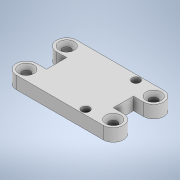
# Autodesk Inventor part: Крепление мотора
Saved by Autodesk Inventor 2020 (Build 240168000, 168)
## iProperties
Created: 2021-05-23
Part Number: Крепление мотора
Material: Типовые
Document SubType Name: Modeling
Designer: Антон
Density: 1 g/cm^3
Appearance: По умолчанию
Author: Антон
Autodesk Inventor part; units mm, degrees
ref_plane "YZ Plane" through (0, 0, 0) normal (1, 0, 0) x (0, 1, 0)
ref_plane "XZ Plane" through (0, 0, 0) normal (0, 1, 0) x (-1, 0, 0)
ref_plane "XY Plane" through (0, 0, 0) normal (0, 0, 1) x (1, 0, 0)
sketch "Эскиз1" plane through (0, 0, 0) normal (0, 1, 0) x (-1, 0, 0)
  line L0 (0, 0) -> (26.5, 0)
  line L1 (26.5, 0) -> (26.5, -24)
  line L2 (26.5, -24) -> (0, -24)
  line L3 (0, -24) -> (0, 0)
  dimension "d0" = 26.5
  dimension "d1" = 24
  constraints: 8 end point, 2 parallel, 1 horizontal, 1 perpendicular
  measures "d0" distance of L1.end L2.end
  measures "d1" distance of L0.end L1.end
extrude "Выдавливание1" add sketch "Эскиз1" along normal blind 5
sketch "Эскиз2" plane through (0, 5, 0) normal (0, 1, 0) x (1, 0, 0)
  line L0 (0, 0) -> (0, 24) projected
  line L1 (0, 12) -> (-5, 12)
  line L2 (-5, 12) -> (-5, 2)
  line L3 (-5, 12) -> (-5, 22)
  dimension "d4" = 5
  dimension "d5" = 10
  constraints: 6 end point, 2 vertical, 1 collinear, 1 midpoint, 1 perpendicular
  measures "d4" distance of L1.start L1.end
  measures "d5" distance of L1.end L2.end
hole "Отверстие1" at (-5, 5, -2) at (-5, 5, -22) direction (0, -1, 0) diameter 3.2 end through all
sketch "Эскиз3" plane through (0, 0, 0) normal (0, -1, 0) x (1, 0, 0)
  line L0 (-26.5, 0) -> (0, 0) projected
  line L1 (0, 0) -> (8, 0)
  line L2 (8, 0) -> (8, -8)
  line L3 (8, -8) -> (0, -8)
  line L4 (0, -8) -> (0, 0)
  dimension "d13" = 8
  dimension "d14" = 8
  constraints: 8 end point, 2 parallel, 1 horizontal, 1 perpendicular
  measures "d13" distance of L2.end L3.end
  measures "d14" distance of L1.end L2.end
extrude "Выдавливание2" add sketch "Эскиз3" against normal blind 5
sketch "Эскиз4" plane through (0, 5, 0) normal (0, 1, 0) x (1, 0, 0)
  line L0 (8, 8) -> (0, 8) projected
  line L1 (4, 8) -> (4, 0)
  point P0 (0, 0)
  point P1 (4, 4)
  constraints: 2 end point, 2 midpoint, 1 vertical
hole "Отверстие2" at (4, 5, -4) direction (0, -1, 0) diameter 3.2 end through all countersink diameter 6 countersink angle 90
fillet "Сопряжение1" radius 4 2 edges at (8, 2.5, 0) (8, 2.5, -8)
ref_plane "РабПлоскость1" through (-26.5, 0, -12) normal (0, 0, 1) x (1, 0, 0)
mirror "Зеркальное отражение1" about plane through (-26.5, 0, -12) normal (0, 0, 1) of "Сопряжение1", "Отверстие2", "Выдавливание2"
ref_plane "РабПлоскость2" through (-13.25, 0, -8) normal (1, 0, 0) x (0, 0, -1)
mirror "Зеркальное отражение2" about plane through (-13.25, 0, -8) normal (1, 0, 0) of "Отверстие2", "Сопряжение1", "Выдавливание2", "Зеркальное отражение1"
